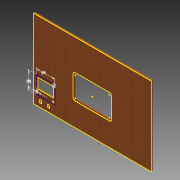
# Autodesk Inventor part: capac cu gaura
Saved by Autodesk Inventor 2015 SP1 (Build 190203100, 203)
## iProperties
Created: 2015-04-26
Part Number: capac cu gaura
Material: Wood (Cherry)
Document SubType Name: Modeling
Designer: ubik
Density: 0.63 g/cm^3
Appearance: Cherry - Natural Low Gloss
Author: ubik
Autodesk Inventor part; units mm, degrees
ref_plane "YZ Plane" through (0, 0, 0) normal (1, 0, 0) x (0, 1, 0)
ref_plane "XZ Plane" through (0, 0, 0) normal (0, 1, 0) x (-1, 0, 0)
ref_plane "XY Plane" through (0, 0, 0) normal (0, 0, 1) x (1, 0, 0)
sketch "Sketch2" plane through (0, 0, 0) normal (0, 0, 1) x (1, 0, 0)
  line L0 (-299.9999, -180.4934) -> (300.0001, -180.4934) projected
  line L1 (300.0001, -180.4934) -> (300.0001, 219.5066) projected
  line L2 (-299.9999, 219.5066) -> (300.0001, 219.5066) projected
  line L3 (-299.9999, -180.4934) -> (-299.9999, 219.5066) projected
  line L4 (-93.75, 46) -> (-93.75, -46) projected
  arc A0 (-93.75, -46) -> (-81.75, -58) centre (-81.75, -46) ccw projected
  line L5 (-81.75, -58) -> (81.75, -58) projected
  arc A1 (81.75, -58) -> (93.75, -46) centre (81.75, -46) ccw projected
  line L6 (93.75, -46) -> (93.75, 46) projected
  arc A2 (93.75, 46) -> (81.75, 58) centre (81.75, 46) ccw projected
  line L7 (81.75, 58) -> (-81.75, 58) projected
  arc A3 (-81.75, 58) -> (-93.75, 46) centre (-81.75, 46) ccw projected
  point P0 (0, 0)
extrude "Extrusion1" add sketch "Sketch2" along normal blind 8
sketch "Sketch3" plane through (0, 0, 8) normal (0, 0, 1) x (1, 0, 0)
  arc A0 (86.75, -63) -> (98.75, -51) centre (86.75, -51) ccw projected
  line L0 (-86.75, -63) -> (86.75, -63) projected
  arc A1 (-98.75, -51) -> (-86.75, -63) centre (-86.75, -51) ccw projected
  line L1 (-98.75, 51) -> (-98.75, -51) projected
  arc A2 (-86.75, 63) -> (-98.75, 51) centre (-86.75, 51) ccw projected
  line L2 (86.75, 63) -> (-86.75, 63) projected
  arc A3 (98.75, 51) -> (86.75, 63) centre (86.75, 51) ccw projected
  line L3 (98.75, -51) -> (98.75, 51) projected
  point P0 (0, 0)
extrude "Extrusion2" cut sketch "Sketch3" against normal blind 4
sketch "Sketch4" plane through (0, 0, 8) normal (0, 0, 1) x (1, 0, 0)
  line L0 (-269.9999, -146.4934) -> (-258.9999, -146.4934)
  line L1 (-258.9999, -146.4934) -> (-258.9999, -160.4934)
  line L2 (-258.9999, -160.4934) -> (-269.9999, -160.4934)
  line L3 (-269.9999, -160.4934) -> (-269.9999, -146.4934)
  line L4 (-228.9999, -146.4934) -> (-217.9999, -146.4934)
  line L5 (-217.9999, -146.4934) -> (-217.9999, -160.4934)
  line L6 (-217.9999, -160.4934) -> (-228.9999, -160.4934)
  line L7 (-228.9999, -160.4934) -> (-228.9999, -146.4934)
  line L8 (-299.9999, 219.5066) -> (-299.9999, -180.4934) projected
  line L9 (-299.9999, -180.4934) -> (300.0001, -180.4934) projected
  line L10 (-299.9999, -131.4934) -> (-6.35, -131.4934) construction
  line L11 (-284.9999, -131.4934) -> (-284.9999, 24.5066) construction
  line L12 (-284.9999, -104.4934) -> (-276.9999, -104.4934) construction
  line L13 (-284.9999, -53.4934) -> (-276.9999, -53.4934) construction
  line L14 (-276.9999, 23.0066) -> (-276.9999, -53.4934) construction
  line L15 (-190.9999, -131.4934) -> (-190.9999, 19.5066) construction
  line L16 (-197.9999, 19.5066) -> (-197.9999, -53.4934) construction
  circle A0 centre (-199.9999, -122.4934) radius 4
  line L17 (-276.9999, -104.4934) -> (-197.9999, -104.4934)
  line L18 (-197.9999, -104.4934) -> (-6.35, -104.4934) construction
  line L19 (-197.9999, -53.4934) -> (-197.9999, -104.4934)
  line L20 (-197.9999, -53.4934) -> (-6.35, -53.4934) construction
  line L21 (-276.9999, -53.4934) -> (-197.9999, -53.4934)
  line L22 (-276.9999, -53.4934) -> (-276.9999, -104.4934)
  line L23 (-276.9999, -104.4934) -> (-276.9999, -131.4934) construction
  point P0 (0, 0)
  dimension "d4" = 30
  dimension "d5" = 20
  dimension "d6" = 14
  dimension "d7" = 11
  dimension "d8" = 30
  dimension "d9" = 11
  dimension "d10" = 15
  dimension "d11" = 15
  dimension "d12" = 27
  dimension "d13" = 51
  dimension "d14" = 8
  dimension "d15" = 94
  dimension "d16" = 79
  dimension "d17" = 8
  dimension "d19" = 85
  dimension "d20" = 9
  constraints: 44 end point, 11 perpendicular, 9 horizontal, 9 point on line, 4 parallel, 2 vertical, 1 centre point, 1 midpoint
  measures "d4" distance between parallel lines of L8 L3
  measures "d5" distance between parallel lines of L9 L2
  measures "d6" distance of L2.end L0.start
  measures "d7" distance of L1.end L2.end
  measures "d8" distance between parallel lines of L7 L1
  measures "d9" distance of L5.end L6.end
  measures "d10" distance between parallel lines of L4 L10
  measures "d11" distance between parallel lines of L8 L11
  measures "d12" distance between parallel lines of L10 L12
  measures "d13" distance between parallel lines of L12 L13
  measures "d14" distance between parallel lines of L11 L14
  measures "d15" distance between parallel lines of L11 L15
  measures "d16" distance between parallel lines of L16 L14
  measures "d17" diameter of A0
  measures "d19" distance from line of L11 A0.centre
  measures "d20" distance from line of L10 A0.centre
extrude "Extrusion3" cut sketch "Sketch4" against normal through all
sketch "Sketch5" plane through (0, 0, 8) normal (0, 0, 1) x (1, 0, 0)
  line L0 (-284.9999, -43.4934) -> (-190.9999, -43.4934)
  line L1 (-190.9999, -43.4934) -> (-190.9999, -131.4934)
  line L2 (-190.9999, -131.4934) -> (-284.9999, -131.4934)
  line L3 (-284.9999, -131.4934) -> (-284.9999, -43.4934)
  line L4 (-276.9999, -104.4934) -> (-276.9999, -53.4934) projected
  line L5 (-276.9999, -53.4934) -> (-197.9999, -53.4934) projected
  line L6 (-217.9999, -160.4934) -> (-217.9999, -146.4934) projected
  line L7 (-217.9999, -146.4934) -> (-228.9999, -146.4934) projected
  line L8 (-228.9999, -146.4934) -> (-228.9999, -160.4934) projected
  line L9 (-228.9999, -160.4934) -> (-217.9999, -160.4934) projected
  circle A0 centre (-199.9999, -122.4934) radius 4 projected
  line L10 (-258.9999, -160.4934) -> (-258.9999, -146.4934) projected
  line L11 (-258.9999, -146.4934) -> (-269.9999, -146.4934) projected
  line L12 (-269.9999, -146.4934) -> (-269.9999, -160.4934) projected
  line L13 (-269.9999, -160.4934) -> (-258.9999, -160.4934) projected
  line L14 (-276.9999, -104.4934) -> (-197.9999, -104.4934) projected
  line L15 (-197.9999, -104.4934) -> (-197.9999, -53.4934) projected
  line L16 (98.75, -51) -> (98.75, 51) projected
  arc A1 (98.75, 51) -> (86.75, 63) centre (86.75, 51) ccw projected
  line L17 (86.75, 63) -> (-86.75, 63) projected
  arc A2 (-86.75, 63) -> (-98.75, 51) centre (-86.75, 51) ccw projected
  line L18 (-98.75, 51) -> (-98.75, -51) projected
  arc A3 (-98.75, -51) -> (-86.75, -63) centre (-86.75, -51) ccw projected
  line L19 (-86.75, -63) -> (86.75, -63) projected
  arc A4 (86.75, -63) -> (98.75, -51) centre (86.75, -51) ccw projected
  line L20 (-299.9999, -180.4934) -> (-299.9999, 219.5066) projected
  line L21 (-299.9999, 219.5066) -> (300.0001, 219.5066) projected
  line L22 (300.0001, 219.5066) -> (300.0001, -180.4934) projected
  line L23 (300.0001, -180.4934) -> (-299.9999, -180.4934) projected
  line L24 (-276.9999, -53.4934) -> (-276.9999, -104.4934) projected
  line L25 (-197.9999, -53.4934) -> (-276.9999, -53.4934) projected
  point P0 (0, 0)
  dimension "d23" = 88
  dimension "d24" = 94
  dimension "d25" = 8
  dimension "d26" = 10
  constraints: 8 end point, 2 parallel, 1 horizontal, 1 perpendicular
  measures "d23" distance of L2.end L0.start
  measures "d24" distance of L0.start L0.end
  measures "d25" distance between parallel lines of L4 L3
  measures "d26" distance between parallel lines of L5 L0
sketch "Sketch6" plane through (0, 0, 0) normal (0, 0, -1) x (-1, 0, 0)
  line L0 (217.9999, -146.4934) -> (217.9999, -160.4934) projected
  line L1 (217.9999, -160.4934) -> (228.9999, -160.4934) projected
  line L2 (228.9999, -160.4934) -> (228.9999, -146.4934) projected
  line L3 (228.9999, -146.4934) -> (217.9999, -146.4934) projected
  circle A0 centre (199.9999, -122.4934) radius 4 projected
  line L4 (258.9999, -146.4934) -> (258.9999, -160.4934) projected
  line L5 (258.9999, -160.4934) -> (269.9999, -160.4934) projected
  line L6 (269.9999, -160.4934) -> (269.9999, -146.4934) projected
  line L7 (269.9999, -146.4934) -> (258.9999, -146.4934) projected
  line L8 (276.9999, -104.4934) -> (276.9999, -53.4934) projected
  line L9 (276.9999, -53.4934) -> (197.9999, -53.4934) projected
  line L10 (197.9999, -53.4934) -> (197.9999, -104.4934) projected
  line L11 (197.9999, -104.4934) -> (276.9999, -104.4934) projected
  arc A1 (-93.75, -46) -> (-81.75, -58) centre (-81.75, -46) ccw projected
  line L12 (-81.75, -58) -> (81.75, -58) projected
  arc A2 (81.75, -58) -> (93.75, -46) centre (81.75, -46) ccw projected
  line L13 (93.75, -46) -> (93.75, 46) projected
  arc A3 (93.75, 46) -> (81.75, 58) centre (81.75, 46) ccw projected
  line L14 (81.75, 58) -> (-81.75, 58) projected
  arc A4 (-81.75, 58) -> (-93.75, 46) centre (-81.75, 46) ccw projected
  line L15 (-93.75, 46) -> (-93.75, -46) projected
  line L16 (299.9999, 219.5066) -> (299.9999, -180.4934) projected
  line L17 (299.9999, -180.4934) -> (-300.0001, -180.4934) projected
  line L18 (-300.0001, -180.4934) -> (-300.0001, 219.5066) projected
  line L19 (-300.0001, 219.5066) -> (299.9999, 219.5066) projected
  line L20 (190.9999, -43.4934) -> (284.9999, -43.4934)
  line L21 (284.9999, -43.4934) -> (284.9999, -131.4934)
  line L22 (284.9999, -131.4934) -> (190.9999, -131.4934)
  line L23 (190.9999, -131.4934) -> (190.9999, -43.4934)
  point P0 (0, 0)
  dimension "d27" = 94
  dimension "d28" = 88
  dimension "d29" = 8
  dimension "d30" = 10
  constraints: 8 end point, 2 parallel, 1 horizontal, 1 perpendicular
  measures "d27" distance of L20.start L20.end
  measures "d28" distance of L22.end L20.start
  measures "d29" distance between parallel lines of L8 L21
  measures "d30" distance between parallel lines of L9 L20
extrude "Extrusion4" cut sketch "Sketch6" against normal blind 3.5 contours L20 L21 L22 L23
equation "\"d9\" = d7"
body "Solid1"
